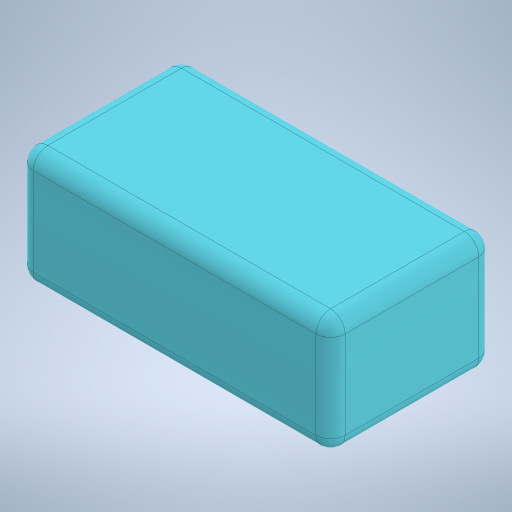
# Autodesk Inventor part: LiPo
Saved by Autodesk Inventor 2024 (Build 280153000, 153)
## iProperties
Created: 2023-10-18
Part Number: LiPo
Material: Generic
Document SubType Name: Modeling
Designer: CJ110
Density: 1 g/cm^3
Appearance: Default
Author: CJ110
Autodesk Inventor part; units mm, degrees
ref_plane "YZ Plane" through (0, 0, 0) normal (1, 0, 0) x (0, 1, 0)
ref_plane "XZ Plane" through (0, 0, 0) normal (0, 1, 0) x (-1, 0, 0)
ref_plane "XY Plane" through (0, 0, 0) normal (0, 0, 1) x (1, 0, 0)
sketch "Sketch1" plane through (0, 0, 0) normal (0, 1, 0) x (-1, 0, 0)
  line L0 (0, 0) -> (68, 0)
  line L1 (68, 0) -> (68, 35.5)
  line L2 (68, 35.5) -> (0, 35.5)
  line L3 (0, 35.5) -> (0, 0)
  dimension "d0" = 35.5
  dimension "d1" = 68
  constraints: 8 end point, 2 parallel, 1 horizontal, 1 perpendicular
  measures "d0" distance of L0.end L1.end
  measures "d1" distance of L1.end L2.end
extrude "Extrusion1" add sketch "Sketch1" along normal blind 25.5
fillet "Fillet1" radius 3.175 12 edges at (-34, 25.5, 35.5) (-34, 25.5, 0) (-34, 0, 0) (-34, 0, 35.5) (0, 25.5, 17.75) (0, 12.75, 35.5) (0, 0, 17.75) (0, 12.75, 0) (-68, 0, 17.75) (-68, 12.75, 35.5) (-68, 25.5, 17.75) (-68, 12.75, 0)
body "Solid1"
